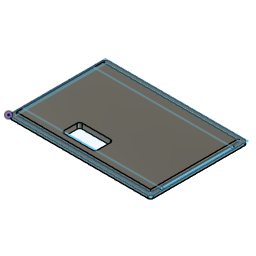
electronics-housing-cover (Autodesk Fusion 360 design; units mm, degrees)
Autodesk Fusion 360 part; units mm, degrees
sketch "Sketch1" plane through (0, 0, 0) normal (0, 0, 1) x (1, 0, 0)
  line L0 (0, 0) -> (110, 0)
  line L1 (110, 0) -> (110, 75)
  line L2 (110, 75) -> (0, 75)
  line L3 (0, 75) -> (0, 0)
  dimension "d1" = 110
  dimension "d2" = 75
  constraint horizontal L0
  constraint vertical L1
  constraint horizontal L2
  constraint vertical L3
  constraint coincident L0.start L3.end
  measures "d1" distance of L0.start L0.end
  measures "d2" distance of L0.start L2.end
extrude "Extrude1" add sketch "Sketch1" along normal blind 2
sketch "Screws" plane through (0, 0, 2) normal (0, 0, 1) x (1, 0, 0)
  line L0 (107, 72) -> (107, 3)
  line L1 (3, 3) -> (3, 72)
  line L2 (3, 72) -> (107, 72)
  line L3 (107, 3) -> (3, 3)
  line L4 (110, 75) -> (0, 75)
  line L5 (0, 0) -> (110, 0)
  line L6 (110, 0) -> (110, 75)
  line L7 (0, 75) -> (0, 0)
  line L8 (1.5, 65) -> (1.5, 10)
  line L9 (108.5, 65) -> (1.5, 65)
  line L10 (1.5, 10) -> (108.5, 10)
  line L11 (108.5, 10) -> (108.5, 65)
  dimension "d10" = 107
  dimension "d12" = 10
  dimension "d13" = 65
  measures "d10" distance of L8.end L10.end
  measures "d12" vertical distance of L5.start L8.end
  measures "d13" vertical distance of L5.start L8.start
hole "Hole1" at (1.5, 10, 2) at (1.5, 65, 2) at (108.5, 65, 2) at (108.5, 10, 2) direction (0, 0, -1) diameter 2 depth 19 tip angle 180
sketch "screw holes" plane through (0, 0, 2) normal (0, 0, 1) x (1, 0, 0)
  line L0 (3, 3) -> (3, 72)
  line L1 (3, 72) -> (107, 72)
  line L2 (107, 72) -> (107, 3)
  line L3 (107, 3) -> (3, 3)
  line L4 (110, 75) -> (0, 75)
  line L5 (0, 0) -> (110, 0)
  line L6 (110, 0) -> (110, 75)
  line L7 (0, 75) -> (0, 0)
  line L8 (1.5, 15) -> (108.5, 15)
  line L9 (108.5, 15) -> (108.5, 65)
  line L10 (1.5, 65) -> (1.5, 15)
  line L11 (108.5, 65) -> (1.5, 65)
extrude "Extrude2" add sketch "screw holes" along normal blind 2 contours L0 L2 L3 L8 | L0 L2 L8 L11 | L0 L1 L2 L11
sketch "Sketch4" plane through (0, 0, 4) normal (0, 0, 1) x (-1, 0, 0)
  line L0 (-107, -3) -> (-107, -72)
  line L1 (-107, -72) -> (-3, -72)
  line L2 (-3, -72) -> (-3, -3)
  line L3 (-3, -3) -> (-107, -3)
  line L4 (-34, -7) -> (-60, -7)
  line L5 (-60, -7) -> (-60, -21)
  line L6 (-60, -21) -> (-34, -21)
  line L7 (-34, -21) -> (-34, -7)
  point P0 (-34, -7)
  dimension "d14" = 7
  dimension "d15" = 34
  dimension "d16" = 60
  dimension "d17" = 21
  constraint horizontal L4
  constraint vertical L5
  constraint horizontal L6
  constraint vertical L7
  constraint coincident P0 L4.start
  measures "d14" vertical distance of P0 origin
  measures "d15" horizontal distance of P0 origin
  measures "d16" distance of origin L5
  measures "d17" distance of origin L6
extrude "Extrude3" cut sketch "Sketch4" against normal blind 5 contours L4 L5 L6 L7
fillet "Fillet1" radius 2 1 edges at (55, 72, 4)
fillet "Fillet1" radius 2 1 edges at (110, 75, 1)
fillet "Fillet1" radius 2 1 edges at (110, 0, 1)
fillet "Fillet1" radius 2 1 edges at (0, 0, 1)
fillet "Fillet1" radius 2 1 edges at (0, 75, 1)
fillet "Fillet1" radius 2 1 edges at (60, 21, 2)
fillet "Fillet1" radius 2 1 edges at (60, 7, 2)
fillet "Fillet1" radius 2 1 edges at (34, 7, 2)
fillet "Fillet1" radius 2 1 edges at (34, 21, 2)
equation "d13 = 75 mm - d12"
